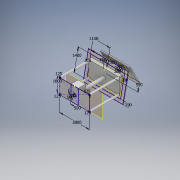
# Autodesk Inventor part: 캡스톤 스테이션 디자인
Saved by Autodesk Inventor 2018 (Build 220112000, 112)
## iProperties
Created: 2021-05-02
Part Number: 캡스톤 스테이션 디자인
Material: 일반
Document SubType Name: Modeling
Designer: ohsm
Density: 1 g/cm^3
Appearance: 기본값
Author: ohsm
Autodesk Inventor part; units mm, degrees
ref_plane "YZ Plane" through (0, 0, 0) normal (1, 0, 0) x (0, 1, 0)
sketch "스케치1" plane through (0, 0, 0) normal (0, 1, 0) x (-1, 0, 0)
  line L0 (-1000, -500) -> (1000, -500)
  line L1 (1000, -500) -> (1000, 500)
  line L2 (1000, 500) -> (-1000, 500)
  line L3 (-1000, 500) -> (-1000, -500)
  line L4 (-1000, -500) -> (1000, 500) construction
  line L5 (1000, -500) -> (-1000, 500) construction
  circle A0 centre (1000, 500) radius 62.5
  circle A1 centre (1000, -500) radius 62.5
  circle A2 centre (-1000, -500) radius 62.5
  circle A3 centre (-1000, 500) radius 62.5
  line L6 (267.7229, 133.8614) -> (-196.5153, -98.2576) construction
  line L7 (-80.4557, 249.921) -> (109.609, -340.4802) construction
  circle A4 centre (0, 0) radius 100
  line L8 (-250, -500) -> (250, -500)
  line L9 (250, -500) -> (250, 500)
  line L10 (250, 500) -> (-250, 500)
  line L11 (-250, 500) -> (-250, -500)
  line L12 (-250, -500) -> (250, 500) construction
  line L13 (250, -500) -> (-250, 500) construction
  point P0 (1000, 0)
  dimension "d0" = 1000
  dimension "d1" = 2000
  dimension "d2" = 125
  dimension "d3" = 125
  dimension "d4" = 125
  dimension "d5" = 125
  dimension "d7" = 500
  dimension "d8" = 200
  dimension "d10" = 500
  constraints: 28 end point, 5 centre point, 5 coincident, 5 midpoint, 4 parallel, 4 point on line, 2 horizontal, 2 perpendicular
  measures "d0" distance of L0.end L1.end
  measures "d1" distance between parallel lines of L3 L1
  measures "d2" diameter of A0
  measures "d3" diameter of A3
  measures "d4" diameter of A2
  measures "d5" diameter of A1
  measures "d7" distance of L7.end L6.start
  measures "d8" diameter of A4
  measures "d10" distance between parallel lines of L11 L9
extrude "돌출1" add sketch "스케치1" along normal blind 2000 contours L3 A2 L0 | L0 A2 L3 | A3 L2 L3 | L3 L2 A3 | A1 L1 L0 | L0 L1 A1 | A0 L1 L2 | L2 L1 A0
extrude "돌출2" add sketch "스케치1" along normal blind 3000 contours A4
extrude "돌출3" add sketch "스케치1" along normal blind 500 contours L11 L2 L9 L0
sketch "스케치2" plane through (-1000, 2000, -500) normal (0, 1, 0) x (1, 0, 0)
  circle A0 centre (2000, -1000) radius 62.5 projected
  line L0 (0, 0) -> (2000, 0)
  line L1 (2000, 0) -> (2000, -1000)
  line L2 (2000, -1000) -> (0, -1000)
  line L3 (0, -1000) -> (0, 0)
  circle A1 centre (0, 0) radius 62.5 projected
  line L4 (-62.5, 62.5) -> (2062.5, 62.5)
  line L5 (2062.5, 62.5) -> (2062.5, -1062.5)
  line L6 (2062.5, -1062.5) -> (-62.5, -1062.5)
  line L7 (-62.5, -1062.5) -> (-62.5, 62.5)
  circle A2 centre (2000, -1000) radius 62.5 projected
  point P0 (1000, -500)
  constraints: 16 end point, 4 parallel, 4 tangent, 2 horizontal, 2 perpendicular, 1 coincident
ref_plane "작업 평면1" through (1000, 2000, -500) normal (0, 1, 0) x (0, 0, 1)
sketch "스케치3" plane through (0, 0, 0) normal (1, 0, 0) x (0, 1, 0)
  line L0 (2000, 437.5) -> (2000, 562.5) projected
  line L1 (2000, 500) -> (2200, 500)
  point P0 (0, 0)
  dimension "d17" = 200
  constraints: 2 end point, 1 horizontal, 1 midpoint
  measures "d17" distance of L1.start L1.end
ref_plane "작업 평면2" through (-1000, 2000, -500) normal (0, -0.9805807, 0.1961161) x (1, 0, 0)
sketch "스케치4" plane through (-1000, 2000, -500) normal (0, -0.9805807, 0.1961161) x (1, 0, 0)
  line L0 (2150, 1236.4065) -> (-150, 1236.4065)
  line L1 (-150, 1236.4065) -> (-150, -163.5935)
  line L2 (-150, -163.5935) -> (2150, -163.5935)
  line L3 (2150, -163.5935) -> (2150, 1236.4065)
  ellipse E0 centre (1000, 686.4065) end of major axis (1100, 686.4065) minor radius 98.0581 projected
  line L4 (1000, 686.4065) -> (1000, 1236.4065)
  line L5 (2350, 1436.4065) -> (-350, 1436.4065)
  line L6 (-350, 1436.4065) -> (-350, -363.5935)
  line L7 (-350, -363.5935) -> (2350, -363.5935)
  line L8 (2350, -363.5935) -> (2350, 1436.4065)
  point P0 (1000, 98.0581)
  dimension "d18" = 2300
  dimension "d19" = 1400
  dimension "d20" = 550
  dimension "d21" = 1150
  dimension "d51" = 200
  dimension "d52" = 200
  dimension "d53" = 200
  dimension "d54" = 200
  constraints: 18 end point, 5 parallel, 3 perpendicular, 2 horizontal, 1 midpoint, 1 other
  measures "d18" distance of L0.start L0.end
  measures "d19" distance of L0.end L1.end
  measures "d20" distance of L4.start L4.end
  measures "d21" distance between parallel lines of L1 L4
  measures "d51" distance between parallel lines of L7 L2
  measures "d52" distance between parallel lines of L0 L5
  measures "d53" distance between parallel lines of L1 L6
  measures "d54" distance between parallel lines of L3 L8
extrude "돌출5" add sketch "스케치4" against normal blind 70 contours E0
extrude "돌출7" add sketch "스케치4" against normal blind 70 contours L3 L2 L1 L0
extrude "돌출9" add sketch "스케치2" along normal up to next contours L5 L6 A0 | A0 L1 L0 A1 L4 L5 | L1 L2 A0 | A0 L2 L3 A1 L0 L1 | L6 L7 A1 L3 L2 A0 | A1 L7 L4 | A1 L3 L0 picked at (1958.6498, -996.3823) picked at (41.3502, -3.6177)
sketch "스케치5" plane through (0, 3000, 0) normal (0, 1, 0) x (1, 0, 0)
  circle A0 centre (0, 0) radius 100
  dimension "d34" = 200
  constraints: 1 centre point, 1 coincident
  measures "d34" diameter of A0
ref_plane "작업 평면4" through (0, 3000, 0) normal (0, 1, 0) x (1, 0, 0)
sketch "스케치6" plane through (0, 3000, 0) normal (0, 1, 0) x (1, 0, 0)
  point P0 (0, 0)
sketch "스케치7" plane through (0, 0, 0) normal (1, 0, 0) x (0, 1, 0)
  point P0 (0, 0)
sketch "스케치8" plane through (0, 0, 0) normal (1, 0, 0) x (0, 1, 0)
  line L0 (3000, -100) -> (3000, 100) projected
  line L1 (3000, 0) -> (2800, 0)
  line L2 (3000, 0) -> (3200, 0)
  point P0 (0, 0)
  dimension "d36" = 200
  constraints: 4 end point, 2 horizontal, 1 midpoint
  measures "d36" distance of L1.start L2.end
sketch "스케치9" plane through (0, 3000, 0) normal (0, 1, 0) x (1, 0, 0)
  line L0 (-100, -100) -> (100, -100)
  line L1 (100, -100) -> (100, 100)
  line L2 (100, 100) -> (-100, 100)
  line L3 (-100, 100) -> (-100, -100)
  line L4 (-100, -100) -> (100, 100) construction
  line L5 (100, -100) -> (-100, 100) construction
  line L6 (100, -100) -> (100, -200)
  point P0 (0, 0)
  dimension "d37" = 200
  dimension "d38" = 200
  dimension "d42" = 100
  constraints: 14 end point, 2 midpoint, 2 parallel, 1 horizontal, 1 perpendicular, 1 vertical
  measures "d37" distance of L2.end L0.start
  measures "d38" distance of L0.start L0.end
  measures "d42" distance of L0.end L6.end
ref_plane "작업 평면5" through (-100, 3000, 100) normal (0, -1, 0) x (1, 0, 0)
ref_plane "작업 평면6" through (0, 3200, 0) normal (0, 0, 1) x (1, 0, 0)
sketch "스케치10" plane through (0, 0, 0) normal (1, 0, 0) x (0, 1, 0)
  line L0 (3000, -100) -> (3000, 100) projected
  line L1 (3000, 0) -> (3200, 0) projected
  line L2 (3100, 0) -> (3000, 200)
  line L3 (3000, 200) -> (3000, 0)
  point P0 (0, 0)
  dimension "d40" = 100
  dimension "d41" = 200
  constraints: 4 end point, 1 midpoint, 1 vertical
  measures "d40" distance from line of L3 L2.start
  measures "d41" distance from line of L1 L2.end
ref_plane "작업 평면7" through (100, 3000, -100) normal (0, -0.4472136, 0.8944272) x (1, 0, 0)
sketch "스케치11" plane through (-1000, 2068.6406, -513.7281) normal (0, 0.9805807, -0.1961161) x (1, 0, 0)
  point P0 (1000, -98.0581)
ref_plane "작업 평면8" through (0, 3100, 0) normal (0, 0.8944272, 0.4472136) x (0, -0.4472136, 0.8944272)
sketch "스케치12" plane through (0, 3100, 0) normal (0, 0.8944272, 0.4472136) x (0, -0.4472136, 0.8944272)
  line L0 (-705.2786, -1000) -> (794.7214, -1000)
  line L1 (794.7214, -1000) -> (794.7214, 1000)
  line L2 (794.7214, 1000) -> (-705.2786, 1000)
  line L3 (-705.2786, 1000) -> (-705.2786, -1000)
  line L4 (44.7214, 937.5) -> (44.7214, -937.5) projected
  line L5 (-705.2786, -1000) -> (794.7214, 1000) construction
  line L6 (794.7214, -1000) -> (-705.2786, 1000) construction
  point P0 (1386.3621, 0)
  point P1 (44.7214, 0)
  dimension "d43" = 1500
  dimension "d44" = 2000
  constraints: 12 end point, 3 midpoint, 2 parallel, 1 horizontal, 1 perpendicular
  measures "d43" distance of L1.end L2.end
  measures "d44" distance between parallel lines of L2 L0
extrude "돌출10" add sketch "스케치12" along normal blind 70
extrude "돌출11" add sketch "스케치9" along normal up to next
extrude "돌출12" add sketch "스케치1" against normal blind 10 contours L3 A2 L0 | A2 L3 A3 L2 L11 L0 | L3 L2 A3 | L9 L2 A0 L1 A1 L0 | A1 L1 L0 | L2 L1 A0 picked at (-962.3809, -482.4579) picked at (-958.6498, 496.3823) picked at (976.1919, -465.9985) picked at (958.6498, 496.3823)
extrude "돌출13" add sketch "스케치4" against normal blind 70 contours L8 L7 L6 L5
sketch "스케치13" plane through (-250, 500, 500) normal (0, 0, 1) x (1, 0, 0)
  point P0 (250, -500)
